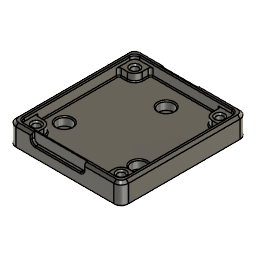
Hub Mount (Autodesk Fusion 360 design; units mm, degrees)
Autodesk Fusion 360 part; units mm, degrees
sketch "Sketch1" plane through (0, 0, 0) normal (0, 0, 1) x (1, 0, 0)
  line L0 (20.5, 23.25) -> (-20.5, 23.25) construction
  line L1 (-20.5, 23.25) -> (-20.5, -23.25) construction
  line L2 (-20.5, -23.25) -> (20.5, -23.25) construction
  line L3 (20.5, -23.25) -> (20.5, 23.25) construction
  line L4 (20.5, 23.25) -> (-20.5, -23.25) construction
  line L5 (-20.5, 23.25) -> (20.5, -23.25) construction
  line L6 (-22.9, -25.65) -> (22.9, -25.65)
  line L7 (22.9, -25.65) -> (22.9, 25.65)
  line L8 (22.9, 25.65) -> (-22.9, 25.65)
  line L9 (-22.9, 25.65) -> (-22.9, -25.65)
  dimension "d2" = 46.5
  dimension "d3" = 41
  dimension "d4" = 2.4
  constraint horizontal L0
  constraint perpendicular L0 L1
  constraint parallel L0 L2
  constraint parallel L1 L3
  constraint coincident L4 origin
  constraint coincident L5 origin
  measures "d2" distance of L0.end L1.end
  measures "d3" distance of L0.start L0.end
extrude "Extrude1" add sketch "Sketch1" along normal blind 8.6
sketch "Sketch2" plane through (0, 0, 8.6) normal (0, 0, 1) x (-1, 0, 0)
  line L0 (22.9, -25.65) -> (22.9, 25.65)
  line L1 (22.9, 25.65) -> (-22.9, 25.65)
  line L2 (-22.9, 25.65) -> (-22.9, -25.65)
  line L3 (-22.9, -25.65) -> (22.9, -25.65)
  line L4 (-17.25, -20) -> (17.25, -20) construction
  line L5 (17.25, -20) -> (17.25, 20) construction
  line L6 (17.25, 20) -> (-17.25, 20) construction
  line L7 (-17.25, 20) -> (-17.25, -20) construction
  line L8 (-17.25, -20) -> (17.25, 20) construction
  line L9 (17.25, -20) -> (-17.25, 20) construction
  circle A0 centre (17.25, 20) radius 1.4
  circle A1 centre (-17.25, 20) radius 1.4
  circle A2 centre (-17.25, -20) radius 1.4
  circle A3 centre (17.25, -20) radius 1.4
  dimension "d7" = 2.8
  dimension "d8" = 40
  dimension "d9" = 34.5
  constraint horizontal L4
  constraint perpendicular L4 L5
  constraint parallel L4 L6
  constraint parallel L5 L7
  constraint coincident L8 origin
  constraint coincident L9 origin
  constraint coincident L5.end L6.start
  constraint coincident L6.end L7.start
  constraint coincident L4.start L7.end
  constraint coincident L4.end L5.start
  constraint equal A0 A1
  constraint equal A1 A2
  constraint equal A2 A3
  measures "d7" diameter of A1
  measures "d8" distance of L4.end L5.end
  measures "d9" distance of L4.start L4.end
extrude "Extrude2" cut sketch "Sketch2" against normal through all contours A0 | A1 | A2 | A3
sketch "Sketch3" plane through (0, 0, 8.6) normal (0, 0, 1) x (-1, 0, 0)
  circle A0 centre (17.25, 20) radius 1.4
  circle A1 centre (-17.25, 20) radius 1.4
  circle A2 centre (17.25, -20) radius 1.4
  circle A3 centre (-17.25, -20) radius 1.4
  line L0 (22.9, -25.65) -> (22.9, 25.65)
  line L1 (22.9, 25.65) -> (-22.9, 25.65)
  line L2 (-22.9, 25.65) -> (-22.9, -25.65)
  line L3 (-22.9, -25.65) -> (22.9, -25.65)
  line L4 (-20.7, -23.45) -> (20.7, -23.45)
  line L5 (20.7, -23.45) -> (20.7, 23.45)
  line L6 (20.7, 23.45) -> (-20.7, 23.45)
  line L7 (-20.7, 23.45) -> (-20.7, -23.45)
  line L8 (-20.7, -23.45) -> (20.7, 23.45) construction
  line L9 (20.7, -23.45) -> (-20.7, 23.45) construction
  dimension "d11" = 2.2
  dimension "d12" = 2.2
  constraint horizontal L4
  constraint perpendicular L4 L5
  constraint parallel L4 L6
  constraint parallel L5 L7
  constraint coincident L8 origin
  constraint coincident L9 origin
  measures "d11" distance of L2 L7
  measures "d12" distance of L3 L4
extrude "Extrude3" cut sketch "Sketch3" against normal blind 1.6 contours L4 L5 L6 L7
fillet "Fillet1" radius 2 4 edges at (-20.7, 23.45, 7.8) (20.7, 23.45, 7.8) (20.7, -23.45, 7.8) (-20.7, -23.45, 7.8)
fillet "Fillet2" radius 3 4 edges at (22.9, 25.65, 4.3) (22.9, -25.65, 4.3) (-22.9, -25.65, 4.3) (-22.9, 25.65, 4.3)
sketch "Sketch4" plane through (0, 0, 7) normal (0, 0, 1) x (-1, 0, 0)
  circle A0 centre (17.25, 20) radius 1.4
  circle A1 centre (-17.25, 20) radius 1.4
  circle A2 centre (-17.25, -20) radius 1.4
  circle A3 centre (17.25, -20) radius 1.4
  arc A4 (20.7, 21.45) -> (18.7, 23.45) centre (18.7, 21.45) ccw
  line L0 (18.7, 23.45) -> (-18.7, 23.45)
  arc A5 (-18.7, 23.45) -> (-20.7, 21.45) centre (-18.7, 21.45) ccw
  line L1 (-20.7, 21.45) -> (-20.7, -21.45)
  arc A6 (-20.7, -21.45) -> (-18.7, -23.45) centre (-18.7, -21.45) ccw
  line L2 (-18.7, -23.45) -> (18.7, -23.45)
  arc A7 (18.7, -23.45) -> (20.7, -21.45) centre (18.7, -21.45) ccw
  line L3 (20.7, -21.45) -> (20.7, 21.45)
  circle A8 centre (17.25, 20) radius 3
  circle A9 centre (-17.25, 20) radius 3
  line L4 (14.25, 20) -> (14.25, 23.45)
  line L5 (17.25, 17) -> (20.7, 17)
  line L6 (-14.25, 20) -> (-14.25, 23.45)
  line L7 (-17.25, 17) -> (-20.7, 17)
  line L8 (0, 0) -> (-20.7, 0) construction
  circle A10 centre (17.25, -20) radius 3
  line L9 (14.25, -20) -> (14.25, -23.45)
  line L10 (17.25, -17) -> (20.7, -17)
  line L11 (-14.25, -20) -> (-14.25, -23.45)
  circle A11 centre (-17.25, -20) radius 3
  line L12 (-17.25, -17) -> (-20.7, -17)
  dimension "d23" = 6
  dimension "d24" = 6
  constraint concentric A0 A8
  constraint concentric A1 A9
  constraint coincident A8 L4.start
  constraint coincident L0 L4.end
  constraint perpendicular L0 L4
  constraint coincident A8 L5.start
  constraint coincident L3 L5.end
  constraint perpendicular L3 L5
  constraint coincident A9 L6.start
  constraint coincident L0 L6.end
  constraint perpendicular L0 L6
  constraint coincident A9 L7.start
  constraint coincident L1 L7.end
  constraint perpendicular L1 L7
  constraint coincident L8.start origin
  constraint midpoint L1 L8.end
  constraint tangent A9 L6
  constraint tangent A9 L7
  constraint tangent A8 L4
  constraint tangent A8 L5
  constraint symmetric A8 L8 A10
  constraint symmetric A9 L8 A11
  constraint symmetric L4.start L8 L9.start
  constraint symmetric L4.end L8 L9.end
  constraint symmetric L5.start L8 L10.start
  constraint symmetric L5.end L8 L10.end
  constraint symmetric L6.start L8 L11.start
  constraint symmetric L6.end L8 L11.end
  constraint symmetric L7.start L8 L12.start
  constraint symmetric L7.end L8 L12.end
  measures "d23" diameter of A9
  measures "d24" diameter of A8
extrude "Extrude4" cut sketch "Sketch4" against normal blind 3 contours L0 L1 L2 L3 A8 A9 L4 L5 L6 L7 A10 L9 L10 L11 A11 L12
fillet "Fillet3" radius 1 8 edges at (-14.25, 23.45, 5.5) (-20.7, 17, 5.5) (14.25, 23.45, 5.5) (20.7, 17, 5.5) (20.7, -17, 5.5) (14.25, -23.45, 5.5) (-14.25, -23.45, 5.5) (-20.7, -17, 5.5)
sketch "Sketch5" plane through (0, 0, 4) normal (0, 0, 1) x (-1, 0, 0)
  arc A0 (20.7, 16) -> (19.7, 17) centre (19.7, 16) ccw
  line L0 (19.7, 17) -> (17.25, 17)
  arc A1 (14.25, 20) -> (17.25, 17) centre (17.25, 20) ccw
  line L1 (14.25, 20) -> (14.25, 22.45)
  arc A2 (14.25, 22.45) -> (13.25, 23.45) centre (13.25, 22.45) ccw
  line L2 (13.25, 23.45) -> (-13.25, 23.45)
  arc A3 (-13.25, 23.45) -> (-14.25, 22.45) centre (-13.25, 22.45) ccw
  line L3 (-14.25, 22.45) -> (-14.25, 20)
  arc A4 (-17.25, 17) -> (-14.25, 20) centre (-17.25, 20) ccw
  line L4 (-17.25, 17) -> (-19.7, 17)
  arc A5 (-19.7, 17) -> (-20.7, 16) centre (-19.7, 16) ccw
  line L5 (-20.7, 16) -> (-20.7, -16)
  arc A6 (-20.7, -16) -> (-19.7, -17) centre (-19.7, -16) ccw
  line L6 (-19.7, -17) -> (-17.25, -17)
  arc A7 (-14.25, -20) -> (-17.25, -17) centre (-17.25, -20) ccw
  line L7 (-14.25, -20) -> (-14.25, -22.45)
  arc A8 (-14.25, -22.45) -> (-13.25, -23.45) centre (-13.25, -22.45) ccw
  line L8 (-13.25, -23.45) -> (13.25, -23.45)
  arc A9 (13.25, -23.45) -> (14.25, -22.45) centre (13.25, -22.45) ccw
  line L9 (14.25, -22.45) -> (14.25, -20)
  arc A10 (17.25, -17) -> (14.25, -20) centre (17.25, -20) ccw
  line L10 (17.25, -17) -> (19.7, -17)
  arc A11 (19.7, -17) -> (20.7, -16) centre (19.7, -16) ccw
  line L11 (20.7, -16) -> (20.7, 16)
  circle A12 centre (0, 2) radius 17.5 construction
  line L12 (0, 0) -> (0, -15.5) construction
  circle A13 centre (0, -15.5) radius 3.05
  line L13 (0, 2) -> (15.1554, 10.75) construction
  line L14 (0, 2) -> (-15.1554, 10.75) construction
  circle A14 centre (15.1554, 10.75) radius 3.05
  circle A15 centre (-15.1554, 10.75) radius 3.05
  line L15 (0, 2) -> (0, 0) construction
  dimension "d25" = 6.1
  dimension "d26" = 120
  dimension "d27" = 120
  dimension "d28" = 6.1
  dimension "d29" = 6.1
  dimension "d30" = 35
  dimension "d50" = 2
  constraint coincident A12.centre L13.start
  constraint coincident A12 L12.end
  constraint vertical L12
  constraint coincident L12.end A13.centre
  constraint coincident A12 L13.end
  constraint coincident A12 L14.end
  constraint coincident L13.end A14.centre
  constraint coincident L14.end A15.centre
  constraint vertical L15
  constraint coincident L12.start L15.end
  measures "d25" diameter of A13
  measures "d26" angle of L12 L14
  measures "d27" angle of L12 L13
  measures "d28" diameter of A14
  measures "d29" diameter of A15
  measures "d30" diameter of A12
  measures "d50" distance of A12.centre L12.start
extrude "Extrude5" cut sketch "Sketch5" against normal blind 3.4 contours A13 | A14 | A15
sketch "Sketch6" plane through (0, 0, 8.6) normal (0, 0, 1) x (-1, 0, 0)
  arc A0 (19.9, -25.65) -> (22.9, -22.65) centre (19.9, -22.65) ccw
  line L0 (22.9, -22.65) -> (22.9, 22.65)
  arc A1 (22.9, 22.65) -> (19.9, 25.65) centre (19.9, 22.65) ccw
  line L1 (19.9, 25.65) -> (-19.9, 25.65)
  arc A2 (-19.9, 25.65) -> (-22.9, 22.65) centre (-19.9, 22.65) ccw
  line L2 (-22.9, 22.65) -> (-22.9, -22.65)
  arc A3 (-22.9, -22.65) -> (-19.9, -25.65) centre (-19.9, -22.65) ccw
  line L3 (-19.9, -25.65) -> (19.9, -25.65)
  line L4 (18.7, -23.45) -> (-18.7, -23.45)
  arc A4 (-20.7, -21.45) -> (-18.7, -23.45) centre (-18.7, -21.45) ccw
  line L5 (-20.7, -21.45) -> (-20.7, 21.45)
  arc A5 (-18.7, 23.45) -> (-20.7, 21.45) centre (-18.7, 21.45) ccw
  line L6 (-18.7, 23.45) -> (18.7, 23.45)
  arc A6 (20.7, 21.45) -> (18.7, 23.45) centre (18.7, 21.45) ccw
  line L7 (20.7, 21.45) -> (20.7, -21.45)
  arc A7 (18.7, -23.45) -> (20.7, -21.45) centre (18.7, -21.45) ccw
  line L8 (10.9, -25.65) -> (-4.1, -25.65)
  line L9 (-4.1, -25.65) -> (-4.1, -24.25)
  line L10 (-4.1, -24.25) -> (10.9, -24.25)
  line L11 (10.9, -24.25) -> (10.9, -25.65)
  line L12 (0, 0) -> (3.4, 0)
  line L13 (3.4, 0) -> (3.4, -24.25) construction
  line L14 (13.7, 25.65) -> (-7.7, 25.65)
  line L15 (-7.7, 25.65) -> (-7.7, 24.25)
  line L16 (-7.7, 24.25) -> (13.7, 24.25)
  line L17 (13.7, 24.25) -> (13.7, 25.65)
  dimension "d34" = 15
  dimension "d35" = 3.4
  dimension "d38" = 0.8
  dimension "d39" = 0.8
  dimension "d41" = 7
  dimension "d42" = 13
  constraint horizontal L8
  constraint vertical L9
  constraint horizontal L10
  constraint vertical L11
  constraint coincident L12.start origin
  constraint horizontal L12
  constraint perpendicular L10 L13
  constraint midpoint L10 L13.end
  constraint collinear L3 L8
  constraint horizontal L14
  constraint vertical L15
  constraint horizontal L16
  constraint vertical L17
  constraint coincident L1 L14.start
  measures "d34" distance of L8.start L8.end
  measures "d35" distance of L12.start L12.end
  measures "d38" distance of L4 L10
  measures "d39" distance of L6 L16
  measures "d41" horizontal distance of A6.start L14.start
  measures "d42" distance of L5 L15
extrude "Extrude6" cut sketch "Sketch6" against normal blind 4 contours L3 L8 L9 L10 L11 | L1 L14 L15 L16 L17
fillet "Fillet4" radius 1.6 4 edges at (-13.7, -24.95, 4.6) (7.7, -24.95, 4.6) (-10.9, 24.95, 4.6) (4.1, 24.95, 4.6)
chamfer "Chamfer1" distance 1 angle 45 10 edges at (22.9, 0, 8.6) (22.0213, 24.7713, 8.6) (12, 25.65, 8.6) (13.8, -25.65, 8.6) (22.0213, -24.7713, 8.6) (-22.0213, 24.7713, 8.6) (-15.4, 25.65, 8.6) (-16.8, -25.65, 8.6) (-22.0213, -24.7713, 8.6) (-22.9, 0, 8.6)
chamfer "Chamfer3" distance 0.6 angle 45 4 edges at (-15.9447, 20.5063, 7) (18.5553, 20.5063, 7) (18.5553, -19.4937, 7) (-15.9447, -19.4937, 7)
chamfer "Chamfer2" distance 0.4 angle 45 45 edges at (0, 23.45, 8.6) (20.1142, 22.8642, 8.6) (20.7, 0, 8.6) (20.1142, -22.8642, 8.6) (0, -23.45, 8.6) (-20.1142, -22.8642, 8.6) (-20.7, 0, 8.6) (-20.1142, 22.8642, 8.6) (-12.3118, -11.8529, 4) (17.999, -11.8529, 4) (2.8436, 14.3971, 4) (20.7, 0, 4) (20.4071, -16.7071, 4) (18.475, -17, 4) (15.1287, -17.8787, 4) (14.25, -21.225, 4) (13.9571, -23.1571, 4) (0, -23.45, 4) (-13.9571, -23.1571, 4) (-14.25, -21.225, 4) (-15.1287, -17.8787, 4) (-18.475, -17, 4) (-20.4071, -16.7071, 4) (-20.7, 0, 4) (-20.4071, 16.7071, 4) (-18.475, 17, 4) (-15.1287, 17.8787, 4) (-14.25, 21.225, 4) (-13.9571, 23.1571, 4) (0, 23.45, 4) (13.9571, 23.1571, 4) (14.25, 21.225, 4) (15.1287, 17.8787, 4) (18.475, 17, 4) (20.4071, 16.7071, 4) (7.2314, -25.65, 5.0686) (7.7, -25.65, 6.9) (-13.7, -25.65, 6.9) (-13.2314, -25.65, 5.0686) (-3, -25.65, 4.6) (3.6314, 25.65, 5.0686) (-3.4, 25.65, 4.6) (-10.4314, 25.65, 5.0686) (-10.9, 25.65, 6.9) (4.1, 25.65, 6.9) 1 faces at (-5.459, -6.3018, 0)
